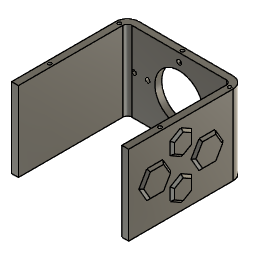
walls2 (Autodesk Fusion 360 design; units mm, degrees)
Autodesk Fusion 360 part; units mm, degrees
note: some values were not read from the file. Set by a fixed rule: which sketch regions a step uses.
sketch "Sketch1" plane through (0, 0, 0) normal (0, 0, 1) x (1, 0, 0)
  line L0 (41.5, 125) -> (-41.5, 125)
  arc A0 (-41.5, 125) -> (-51.5, 115) centre (-41.5, 115) ccw
  line L1 (-51.5, 115) -> (-51.5, -130)
  arc A1 (51.5, 115) -> (41.5, 125) centre (41.5, 115) ccw
  line L2 (51.5, -130) -> (51.5, 115)
  line L3 (-41.5, -140) -> (41.5, -140)
  arc A2 (41.5, -140) -> (51.5, -130) centre (41.5, -130) ccw
  arc A3 (-51.5, -130) -> (-41.5, -140) centre (-41.5, -130) ccw
  line L4 (0, 125) -> (0, 122)
  line L5 (-51.5, 115) -> (-48.5, 115)
  circle A4 centre (-48.5, 115) radius 1.5
  circle A5 centre (0, 122) radius 1.5
  circle A6 centre (-48.5, -7.5) radius 1.5
  circle A7 centre (-48.5, 53.75) radius 1.5
  circle A8 centre (-48.5, -130) radius 1.5
  circle A9 centre (-48.5, -68.75) radius 1.5
  circle A10 centre (-48.5, -7.5) radius 1.5
  circle A11 centre (48.5, 115) radius 1.5
  circle A12 centre (48.5, 53.75) radius 1.5
  circle A13 centre (48.5, -7.5) radius 1.5
  circle A14 centre (48.5, -68.75) radius 1.5
  circle A15 centre (48.5, -130) radius 1.5
  line L6 (0, -140) -> (0, -137)
  circle A16 centre (0, -137) radius 1.5
  arc A17 (-45.5, -130) -> (-41.5, -134) centre (-41.5, -130) ccw
  line L7 (-41.5, -134) -> (41.5, -134)
  arc A18 (41.5, -134) -> (45.5, -130) centre (41.5, -130) ccw
  arc A19 (45.5, 115) -> (41.5, 119) centre (41.5, 115) ccw
  line L8 (41.5, 119) -> (-41.5, 119)
  line L9 (-48.5, -99.375) -> (-48.5, -75)
  line L10 (-48.5, -99.375) -> (-48.5, -125)
  line L11 (-45.5, 115) -> (-45.5, -75)
  line L12 (-45.5, -125) -> (-45.5, -130)
  line L13 (45.5, -130) -> (45.5, -125)
  line L14 (45.5, -75) -> (45.5, 115)
  line L15 (-48.5, -75) -> (-45.5, -75)
  line L16 (45.5, -75) -> (48.5, -75)
  line L17 (-48.5, -125) -> (-45.5, -125)
  line L18 (45.5, -125) -> (48.5, -125)
  line L19 (-48.5, -75) -> (-48.5, -125)
  line L20 (48.5, -75) -> (48.5, -125)
  arc A20 (-41.5, 119) -> (-45.5, 115) centre (-41.5, 115) ccw
  dimension "d1" = 3
  dimension "d3" = 3
  dimension "d4" = 3
  dimension "d5" = 3
  dimension "d7" = 3
  dimension "d8" = 3
  dimension "d9" = 3
  dimension "d10" = 3
  constraint midpoint L0 L4.start
  constraint perpendicular L0 L4
  constraint coincident L5.end A4.centre
  constraint coincident L4.end A5.centre
  constraint symmetric L4 A4 A11
  constraint symmetric L4 A7 A12
  constraint symmetric L4 A8 A15
  constraint symmetric L4 A9 A14
  constraint symmetric L4 A10 A13
  constraint midpoint L3 L6.start
  constraint perpendicular L3 L6
  constraint coincident L6.end A16.centre
  constraint perpendicular L10 L15
  constraint concentric A3 A17
  constraint concentric A2 A18
  constraint concentric A1 A19
  constraint tangent L7 A18
  constraint tangent A17 L7
  constraint tangent A17 L11
  constraint tangent A19 L13
  constraint tangent A18 L13
  constraint tangent A19 L8
  constraint collinear L11 L12
  constraint coincident L13.end L17
  constraint coincident L14.start L15
  constraint collinear L13 L14
  constraint collinear L15 L16
  constraint collinear L17 L18
  constraint symmetric L4 A19.start L11.start
  constraint symmetric L4 A19.end L8.end
  constraint symmetric L4 A19 A20
  measures "d1" distance of L4.start L4.end
  measures "d3" distance of A0.end L5.end
  measures "d4" diameter of A4
  measures "d5" diameter of A5
  measures "d7" diameter of A6
  measures "d8" diameter of A7
  measures "d9" distance of L6.start L6.end
  measures "d10" diameter of A16
extrude "Extrude1" add sketch "Sketch1" along normal blind 70
fillet "Fillet1" radius 5 4 edges at (45.5, -125, 35) (45.5, -75, 35) (-45.5, -75, 35) (-45.5, -125, 35)
sketch "Sketch2" plane through (0, 0, 70) normal (0, 0, 1) x (-1, 0, 0)
  arc A0 (45.5, 129.5826) -> (48.5, 125) centre (50.5, 129.5826) ccw
  line L0 (48.5, 125) -> (48.5, 75)
  arc A1 (48.5, 75) -> (45.5, 70.4174) centre (50.5, 70.4174) ccw
  line L1 (45.5, 70.4174) -> (45.5, -115)
  arc A2 (41.5, -119) -> (45.5, -115) centre (41.5, -115) ccw
  line L2 (41.5, -119) -> (-41.5, -119)
  arc A3 (-45.5, -115) -> (-41.5, -119) centre (-41.5, -115) ccw
  line L3 (-45.5, -115) -> (-45.5, 70.4174)
  arc A4 (-45.5, 70.4174) -> (-48.5, 75) centre (-50.5, 70.4174) ccw
  line L4 (-48.5, 75) -> (-48.5, 125)
  arc A5 (-48.5, 125) -> (-45.5, 129.5826) centre (-50.5, 129.5826) ccw
  line L5 (-45.5, 129.5826) -> (-45.5, 130)
  arc A6 (-41.5, 134) -> (-45.5, 130) centre (-41.5, 130) ccw
  line L6 (-41.5, 134) -> (41.5, 134)
  arc A7 (45.5, 130) -> (41.5, 134) centre (41.5, 130) ccw
  line L7 (45.5, 130) -> (45.5, 129.5826)
  circle A8 centre (48.5, -115) radius 1.5
  circle A9 centre (0, 137) radius 1.5
  circle A10 centre (0, -122) radius 1.5
  circle A11 centre (-48.5, 68.75) radius 1.5
  circle A12 centre (48.5, 130) radius 1.5
  circle A13 centre (-48.5, -115) radius 1.5
  circle A14 centre (-48.5, 130) radius 1.5
  circle A15 centre (48.5, 7.5) radius 1.5
  circle A16 centre (48.5, -53.75) radius 1.5
  circle A17 centre (-48.5, -53.75) radius 1.5
  circle A18 centre (-48.5, 7.5) radius 1.5
  circle A19 centre (48.5, 68.75) radius 1.5
  arc A20 (51.5, 130) -> (41.5, 140) centre (41.5, 130) ccw
  line L8 (41.5, 140) -> (-41.5, 140)
  arc A21 (-41.5, 140) -> (-51.5, 130) centre (-41.5, 130) ccw
  line L9 (-51.5, 130) -> (-51.5, -115)
  arc A22 (-51.5, -115) -> (-41.5, -125) centre (-41.5, -115) ccw
  line L10 (-41.5, -125) -> (41.5, -125)
  arc A23 (41.5, -125) -> (51.5, -115) centre (41.5, -115) ccw
  line L11 (51.5, -115) -> (51.5, 130)
  line L12 (48.5, -53.75) -> (48.5, 7.5)
  line L13 (-48.5, -53.75) -> (-48.5, 7.5)
  line L14 (48.5, -23.125) -> (-48.5, -23.125)
  line L15 (51.5, -23.125) -> (48.5, -23.125)
  line L16 (-48.5, -23.125) -> (-56, -23.125)
  constraint coincident A16.centre L12.start
  constraint coincident A15.centre L12.end
  constraint coincident A17.centre L13.start
  constraint coincident A18.centre L13.end
  constraint midpoint L12 L14.start
  constraint midpoint L13 L14.end
  constraint coincident L11 L15.start
  constraint perpendicular L12 L15
  constraint perpendicular L9 L16
extrude "Extrude2" cut sketch "Sketch2" against normal blind 80 contours A0 L0 A1 L1 L3 A4 L4 A5 L5 A6 L6 A7 L7 A20 L8 A21 L9 L11 L14 L15 L16
sketch "Sketch3" plane through (0, 125, 0) normal (0, 1, 0) x (-1, 0, 0)
  line L0 (-41.5, 0) -> (41.5, 0)
  line L1 (41.5, 0) -> (41.5, 70)
  line L2 (41.5, 70) -> (-41.5, 70)
  line L3 (-41.5, 70) -> (-41.5, 0)
  line L4 (0, 70) -> (0, 0)
  line L5 (0, 35) -> (-16.6685, 35)
  line L6 (2, 37) -> (2, 56.1557)
  arc A0 (2, 13.8443) -> (21.1557, 33) centre (0, 35) ccw
  arc A1 (-2, 56.1557) -> (-21.1557, 37) centre (0, 35) ccw
  line L7 (21.1557, 37) -> (2, 37)
  line L8 (-2, 33) -> (-2, 13.8443)
  line L9 (2, 33) -> (21.1557, 33)
  line L10 (-21.1557, 33) -> (-2, 33)
  circle A2 centre (0, 35) radius 32.5
  line L11 (-2, 37) -> (-21.1557, 37)
  circle A3 centre (0, 7.375) radius 2
  arc A4 (-21.1557, 33) -> (-2, 13.8443) centre (0, 35) ccw
  circle A5 centre (0, 62.625) radius 2
  line L12 (-2, 56.1557) -> (-2, 37)
  line L13 (2, 13.8443) -> (2, 33)
  circle A6 centre (27.625, 35) radius 2
  circle A7 centre (-27.625, 35) radius 2
  arc A8 (21.1557, 37) -> (2, 56.1557) centre (0, 35) ccw
  line L14 (-27.625, 35) -> (-39.625, 35)
  circle A9 centre (-39.625, 35) radius 2
  line L15 (27.625, 35) -> (39.625, 35)
  circle A10 centre (39.625, 35) radius 2
  circle A11 centre (0, 35) radius 21.25
  point P0 (0, 35)
  dimension "d18" = 12
  dimension "d19" = 4
  dimension "d20" = 12
  dimension "d21" = 4
  constraint midpoint L2 L4.start
  constraint coincident L4.end origin
  constraint midpoint L4 P0
  constraint perpendicular L4 L5
  constraint coincident A7.centre L14.start
  constraint perpendicular L3 L14
  constraint coincident L14.end A9.centre
  constraint coincident A6.centre L15.start
  constraint horizontal L15
  constraint coincident L15.end A10.centre
  constraint coincident P0 L5.start
  measures "d18" distance of A7.centre L14.end
  measures "d19" diameter of A9
  measures "d20" distance of A6.centre L15.end
  measures "d21" diameter of A10
extrude "Extrude3" cut sketch "Sketch3" against normal blind 10 contours L3 A9 | L1 A10 | L4 A3 | L4 A3 | L4 L8 L10 L11 L12 A11 | L4 L6 L7 L9 L13 A11 | L4 A5 | L4 A5 | L8 L10 A4 A11 | A0 L9 L13 A11 | L6 L7 A8 A11 | A1 L11 L12 A11 | A6 | A7 picked at (-40.0166, 34.7473) picked at (40.429, 35.5515)
sketch "Sketch4" plane through (51.5, 0, 0) normal (1, 0, 0) x (0, 1, 0)
  line L0 (23.125, 70) -> (23.125, 0)
  line L1 (23.125, 0) -> (115, 0)
  line L2 (115, 0) -> (115, 70)
  line L3 (115, 70) -> (23.125, 70)
  line L4 (69.0625, 70) -> (69.0625, 0)
  line L5 (23.125, 35) -> (69.0625, 35)
  line L6 (69.0625, 70) -> (69.0625, 35)
  line L7 (69.0625, 41.5) -> (78.5888, 47)
  line L8 (78.5888, 47) -> (78.5888, 58)
  line L9 (78.5888, 58) -> (69.0625, 63.5)
  line L10 (69.0625, 63.5) -> (59.5362, 58)
  line L11 (59.5362, 58) -> (59.5362, 47)
  line L12 (59.5362, 47) -> (69.0625, 41.5)
  line L13 (59.5362, 12) -> (59.5362, 23)
  line L14 (69.0625, 6.5) -> (59.5362, 12)
  line L15 (78.5888, 12) -> (69.0625, 6.5)
  line L16 (78.5888, 23) -> (78.5888, 12)
  line L17 (69.0625, 28.5) -> (78.5888, 23)
  line L18 (59.5362, 23) -> (69.0625, 28.5)
  line L19 (32.0937, 35) -> (39.0937, 22.8756)
  line L20 (39.0937, 22.8756) -> (53.0937, 22.8756)
  line L21 (53.0937, 22.8756) -> (60.0937, 35)
  line L22 (60.0937, 35) -> (53.0937, 47.1244)
  line L23 (53.0937, 47.1244) -> (39.0937, 47.1244)
  line L24 (39.0937, 47.1244) -> (32.0937, 35)
  line L25 (85.0312, 47.1244) -> (99.0312, 47.1244)
  line L26 (99.0312, 47.1244) -> (106.0312, 35)
  line L27 (106.0312, 35) -> (99.0312, 22.8756)
  line L28 (99.0312, 22.8756) -> (85.0312, 22.8756)
  line L29 (85.0312, 22.8756) -> (78.0312, 35)
  line L30 (78.0312, 35) -> (85.0312, 47.1244)
  point P0 (69.0625, 52.5)
  point P1 (46.0937, 35)
  dimension "d24" = 11
  dimension "d25" = 14
  constraint midpoint L3 L4.start
  constraint midpoint L1 L4.end
  constraint midpoint L0 L5.start
  constraint midpoint L4 L5.end
  constraint midpoint L6 P0
  constraint symmetric L5 L7.start L17.start
  constraint symmetric L5 L7.end L16.start
  constraint symmetric L5 L8.end L15.start
  constraint symmetric L5 L9.end L14.start
  constraint symmetric L5 L10.end L13.start
  constraint symmetric L5 L11.end L13.end
  constraint midpoint L5 P1
  constraint symmetric L6 L19.start L26.end
  constraint symmetric L6 L19.end L27.end
  constraint symmetric L6 L20.end L28.end
  constraint symmetric L6 L21.end L29.end
  constraint symmetric L6 L22.end L25.start
  constraint symmetric L6 L23.end L25.end
  measures "d24" distance of L7.start P0
  measures "d25" distance of L19.start P1
extrude "Extrude4" add sketch "Sketch4" along normal blind 2 contours L5 L22 L23 L24 | L5 L19 L20 L21 | L4 L6 L7 L8 L9 | L4 L6 L10 L11 L12 | L4 L13 L14 L18 | L4 L15 L16 L17 | L25 L26 L27 L28 L29 L30
chamfer "Chamfer1" distance 2 angle 45 24 edges at (53.5, 46.0937, 47.1244) (53.5, 35.5937, 41.0622) (53.5, 35.5937, 28.9378) (53.5, 56.5937, 41.0622) (53.5, 81.5312, 41.0622) (53.5, 92.0312, 47.1244) (53.5, 102.5312, 41.0622) (53.5, 102.5312, 28.9378) (53.5, 92.0312, 22.8756) (53.5, 81.5312, 28.9378) (53.5, 56.5937, 28.9378) (53.5, 46.0937, 22.8756) (53.5, 64.2994, 25.75) (53.5, 73.8256, 25.75) (53.5, 78.5888, 17.5) (53.5, 73.8256, 9.25) (53.5, 64.2994, 9.25) (53.5, 59.5362, 17.5) (53.5, 64.2994, 60.75) (53.5, 73.8256, 60.75) (53.5, 78.5888, 52.5) (53.5, 73.8256, 44.25) (53.5, 64.2994, 44.25) (53.5, 59.5362, 52.5)
sketch "Sketch6" plane through (-51.5, 0, 0) normal (-1, 0, 0) x (0, -1, 0)
  line L0 (-23.125, 0) -> (-23.125, 70)
  line L1 (-23.125, 70) -> (-115, 70)
  line L2 (-115, 70) -> (-115, 0)
  line L3 (-115, 0) -> (-23.125, 0)
  line L4 (-59.5362, 47) -> (-69.0625, 41.5)
  line L5 (-69.0625, 41.5) -> (-78.5888, 47)
  line L6 (-78.5888, 47) -> (-78.5888, 58)
  line L7 (-78.5888, 58) -> (-69.0625, 63.5)
  line L8 (-69.0625, 63.5) -> (-59.5362, 58)
  line L9 (-59.5362, 58) -> (-59.5362, 47)
  line L10 (-60.0937, 35) -> (-53.0937, 47.1244)
  line L11 (-53.0937, 47.1244) -> (-39.0937, 47.1244)
  line L12 (-39.0937, 47.1244) -> (-32.0937, 35)
  line L13 (-32.0937, 35) -> (-39.0937, 22.8756)
  line L14 (-39.0937, 22.8756) -> (-53.0937, 22.8756)
  line L15 (-53.0937, 22.8756) -> (-60.0937, 35)
  line L16 (-59.5362, 23) -> (-69.0625, 28.5)
  line L17 (-59.5362, 12) -> (-59.5362, 23)
  line L18 (-69.0625, 6.5) -> (-59.5362, 12)
  line L19 (-78.5888, 12) -> (-69.0625, 6.5)
  line L20 (-78.5888, 23) -> (-78.5888, 12)
  line L21 (-69.0625, 28.5) -> (-78.5888, 23)
  line L22 (-99.0312, 22.8756) -> (-85.0312, 22.8756)
  line L23 (-78.0312, 35) -> (-85.0312, 47.1244)
  line L24 (-85.0312, 22.8756) -> (-78.0312, 35)
  line L25 (-85.0312, 47.1244) -> (-99.0312, 47.1244)
  line L26 (-99.0312, 47.1244) -> (-106.0312, 35)
  line L27 (-106.0312, 35) -> (-99.0312, 22.8756)
extrude "Extrude5" add sketch "Sketch6" along normal blind 2 contours L4 L5 L6 L7 L8 L9 | L10 L11 L12 L13 L14 L15 | L16 L17 L18 L19 L20 L21 | L22 L23 L24 L25 L26 L27
chamfer "Chamfer2" distance 2 angle 45 24 edges at (-53.5, 73.8256, 60.75) (-53.5, 64.2994, 60.75) (-53.5, 59.5362, 52.5) (-53.5, 64.2994, 44.25) (-53.5, 73.8256, 44.25) (-53.5, 78.5888, 52.5) (-53.5, 92.0312, 47.1244) (-53.5, 81.5312, 41.0622) (-53.5, 81.5312, 28.9378) (-53.5, 92.0312, 22.8756) (-53.5, 102.5312, 28.9378) (-53.5, 102.5312, 41.0622) (-53.5, 73.8256, 25.75) (-53.5, 64.2994, 25.75) (-53.5, 59.5362, 17.5) (-53.5, 64.2994, 9.25) (-53.5, 73.8256, 9.25) (-53.5, 78.5888, 17.5) (-53.5, 56.5937, 41.0622) (-53.5, 46.0937, 47.1244) (-53.5, 35.5937, 41.0622) (-53.5, 35.5937, 28.9378) (-53.5, 46.0937, 22.8756) (-53.5, 56.5937, 28.9378)
